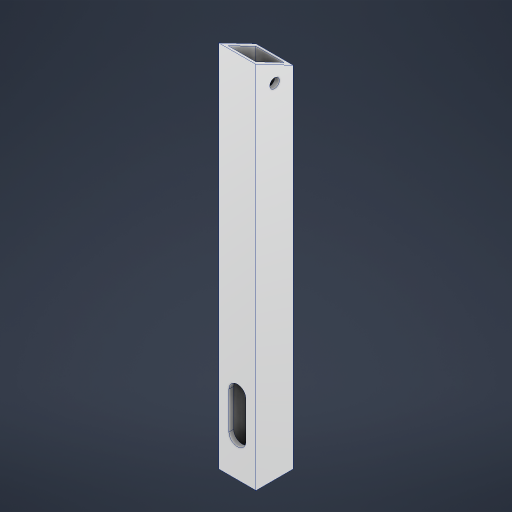
# Autodesk Inventor part: STRU_014_BilletPole_9in_Angled
Saved by Autodesk Inventor 2024.2 (Build 282272000, 272)
## iProperties
Created: 2024-07-25
Part Number: STRU_014_BilletPole_9in_Angled
Material: Aluminum 6061
Document SubType Name: Modeling
Designer: Bryan
Density: 2.7 g/cm^3
Appearance: Aluminum - Flat
Author: Bryan
Autodesk Inventor part; units mm, degrees
ref_plane "YZ Plane" through (0, 0, 0) normal (1, 0, 0) x (0, 1, 0)
ref_plane "XZ Plane" through (0, 0, 0) normal (0, 1, 0) x (-1, 0, 0)
ref_plane "XY Plane" through (0, 0, 0) normal (0, 0, 1) x (1, 0, 0)
sketch "Sketch1" plane through (0, 0, 0) normal (0, 1, 0) x (-1, 0, 0)
  line L0 (-12.7, -12.7) -> (12.7, -12.7)
  line L1 (12.7, -12.7) -> (12.7, 12.7)
  line L2 (12.7, 12.7) -> (-12.7, 12.7)
  line L3 (-12.7, 12.7) -> (-12.7, -12.7)
  line L4 (-12.7, -12.7) -> (12.7, 12.7) construction
  line L5 (12.7, -12.7) -> (-12.7, 12.7) construction
  line L6 (9.525, 9.525) -> (9.525, -9.525)
  line L7 (9.525, -9.525) -> (-9.525, -9.525)
  line L8 (-9.525, -9.525) -> (-9.525, 9.525)
  line L9 (-9.525, 9.525) -> (9.525, 9.525)
  point P0 (0, 0)
  dimension "d0" = 25.4
  dimension "d1" = 25.4
  dimension "d2" = 3.175
  constraints: 20 end point, 4 parallel, 2 midpoint, 2 perpendicular, 1 horizontal, 3 other
  measures "d0" distance of L2.end L1.end
  measures "d1" distance of L1.end L0.end
  measures "d2" distance between parallel lines of L1 L6
extrude "Extrusion1" add sketch "Sketch1" along normal blind 252.3942
sketch "Sketch2" plane through (12.7, 0, 12.7) normal (1, 0, 0) x (0, 0, -1)
  line L0 (0, 0) -> (25.4, 0) projected
  line L1 (25.4, 0) -> (25.4, 252.3942) projected
  line L2 (0, 252.3942) -> (25.4, 252.3942) projected
  line L3 (0, 0) -> (0, 252.3942) projected
  line L4 (0, 252.3942) -> (25.4, 239.2235)
  point P0 (12.7, 0)
  dimension "d5" = 27.408
  constraints: 2 end point, 1 point on line
  measures "d5" angle of L2 L4
extrude "Extrusion2" cut sketch "Sketch2" against normal blind 252.3942 contours L2 L1 L4
sketch "Sketch3" plane through (12.7, 0, 12.7) normal (1, 0, 0) x (0, 0, -1)
  line L0 (0, 252.3942) -> (25.4, 239.2235) construction
  line L1 (0, 252.3942) -> (0, 266.7) construction
  line L2 (25.4, 239.2235) -> (25.4, 266.7) construction
  line L3 (25.4, 266.7) -> (0, 266.7) construction
  line L4 (25.4, 292.1) -> (0, 292.1) construction
  line L5 (0, 292.1) -> (0, 266.7) construction
  line L6 (0, 266.7) -> (25.4, 266.7) construction
  line L7 (25.4, 266.7) -> (25.4, 292.1) construction
  line L8 (25.4, 292.1) -> (0, 266.7) construction
  line L9 (0, 292.1) -> (25.4, 266.7) construction
  circle A0 centre (12.7, 257.175) radius 3.2512 construction
  circle A1 centre (12.7, 279.4) radius 2.4892 construction
  circle A2 centre (12.7, 234.95) radius 3.2512
  point P0 (12.7, 0)
  dimension "d8" = 14.3058
  dimension "d9" = 25.4
  dimension "d10" = 25.4
  dimension "d11" = 6.5024
  dimension "d12" = 4.9784
  dimension "d13" = 22.225
  dimension "d14" = 22.225
  constraints: 18 end point, 3 centre point, 2 horizontal, 2 midpoint, 2 parallel, 2 vertical, 2 vertical alignment, 1 coincident, 1 equal radius, 1 perpendicular
  measures "d8" distance of L0.start L1.end
  measures "d9" distance of L1.end L6.end
  measures "d10" distance of L1.end L4.end
  measures "d11" diameter of A0
  measures "d12" diameter of A1
  measures "d13" distance of point (12.7, 279.4) A0.centre
  measures "d14" distance of A0.centre A2.centre
extrude "Extrusion3" cut sketch "Sketch3" against normal through all
sketch "Sketch4" plane through (12.7, 0, -12.7) normal (0, 0, -1) x (-1, 0, 0)
  circle A0 centre (12.7, 25.4) radius 3.2512
  circle A1 centre (12.7, 50.8) radius 3.2512
  line L0 (0, 0) -> (25.4, 0) projected
  point P0 (12.7, 0)
  point P1 (12.7, 0)
  point P2 (12.7, 0)
  dimension "d17" = 6.5024
  dimension "d18" = 6.5024
  dimension "d19" = 25.4
  dimension "d20" = 25.4
  constraints: 2 centre point, 2 midpoint, 2 vertical alignment
  measures "d17" diameter of A0
  measures "d18" diameter of A1
  measures "d19" distance of point (12.7, 0) A0.centre
  measures "d20" distance of A0.centre A1.centre
extrude "Extrusion4" cut sketch "Sketch4" against normal blind 25.4
sketch "Sketch5" plane through (-12.7, 0, 12.7) normal (0, 0, 1) x (1, 0, 0)
  circle A0 centre (12.7, 25.4) radius 3.2512 construction
  circle A1 centre (12.7, 50.8) radius 3.2512 construction
  line L0 (15.9512, 25.4) -> (15.9512, 50.8) construction
  line L1 (9.4488, 25.4) -> (9.4488, 50.8) construction
  arc A2 (9.4488, 25.4) -> (15.9512, 25.4) centre (12.7, 25.4) ccw construction
  arc A3 (15.9512, 50.8) -> (9.4488, 50.8) centre (12.7, 50.8) ccw construction
  line L2 (18.4912, 50.8) -> (18.4912, 25.4)
  arc A4 (6.9088, 25.4) -> (18.4912, 25.4) centre (12.7, 25.4) ccw
  line L3 (6.9088, 25.4) -> (6.9088, 50.8)
  arc A5 (18.4912, 50.8) -> (6.9088, 50.8) centre (12.7, 50.8) ccw
  point P0 (12.7, 0)
  dimension "d26" = 2.54
  constraints: 12 point on circle, 8 end point, 8 tangent, 4 centre point, 3 other
  measures "d26" distance between parallel lines of L0 L2
extrude "Extrusion5" cut sketch "Sketch5" against normal blind 3.175
body "Solid1"
